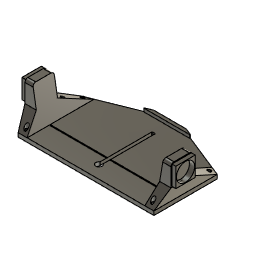
openastrotracker-cameramount (Autodesk Fusion 360 design; units mm, degrees)
Autodesk Fusion 360 part; units mm, degrees
note: some values were not read from the file. Chosen so that the rebuilt part matches the saved one: which bodies a step acts on; which pieces of a blend or face edit are solid.
sketch "Sketch1" plane through (0, 0, 0) normal (0, 1, 0) x (1, 0, 0)
  line L0 (145.5, -42) -> (-145.5, -42)
  line L1 (-145.5, -42) -> (-145.5, 42)
  line L2 (-145.5, 42) -> (145.5, 42)
  line L3 (145.5, 42) -> (145.5, -42)
  line L4 (145.5, -42) -> (-145.5, 42) construction
  line L5 (-145.5, -42) -> (145.5, 42) construction
  dimension "d1" = 291
  dimension "d2" = 84
  constraint perpendicular L0 L1
  constraint parallel L0 L2
  constraint parallel L1 L3
  constraint horizontal L0
  constraint coincident L4 origin
  constraint coincident L5 origin
  measures "d1" distance of L1.end L2.end
  measures "d2" distance of L0.end L1.end
  measures "d167" distance of L0.start
ref_plane "WorkPlane2" through (0, 0, -42) normal (0, 0, 1) x (1, 0, 0)
sketch "Sketch15" plane through (0, 0, -42) normal (0, 0, 1) x (1, 0, 0)
  line L0 (105, 0) -> (105, 95)
  line L1 (105, 95) -> (0, 95)
  line L2 (-105, 0) -> (-105, 95)
  line L3 (-105, 95) -> (0, 95)
  line L4 (105, 0) -> (105, -35)
  line L5 (105, -35) -> (0, -35)
  line L6 (-105, 0) -> (-105, -35)
  line L7 (-105, -35) -> (0, -35)
  line L8 (105, 70) -> (-105, 70)
  line L9 (-105, -20) -> (105, -20)
  line L10 (2.5, 95) -> (-2.5, 95)
  line L11 (-2.5, 95) -> (-2.5, -35)
  line L12 (-2.5, -35) -> (2.5, -35)
  line L13 (2.5, -35) -> (2.5, 95)
  line L14 (2.5, 95) -> (-2.5, -35) construction
  line L15 (-2.5, 95) -> (2.5, -35) construction
  circle A0 centre (0, -15) radius 5
  line L16 (-105, 95) -> (105, 95)
  line L17 (105, 95) -> (105, 90)
  line L18 (105, 90) -> (-105, 90)
  line L19 (-105, 90) -> (-105, 95)
  line L20 (105, 95) -> (-105, 95)
  line L21 (-105, 95) -> (-105, 63)
  line L22 (-105, 63) -> (105, 63)
  line L23 (105, 63) -> (105, 95)
  line L24 (105, 63) -> (25, 95)
  line L25 (-25, 95) -> (-105, 63)
  point P0 (0, 30)
  point P1 (0, 30)
  dimension "d64" = 105
  dimension "d65" = 95
  dimension "d66" = 105
  dimension "d67" = 95
  dimension "d68" = 105
  dimension "d69" = 35
  dimension "d70" = 105
  dimension "d71" = 35
  dimension "d72" = 25
  dimension "d73" = 15
  dimension "d76" = 130
  dimension "d77" = 5
  dimension "d78" = 10
  dimension "d79" = 5
  dimension "d160" = 32
  constraint vertical L0
  constraint horizontal L1
  constraint vertical L2
  constraint horizontal L3
  constraint vertical L4
  constraint horizontal L5
  constraint vertical L6
  constraint horizontal L7
  constraint coincident L0 L8.start
  constraint coincident L2 L8.end
  constraint perpendicular L2 L8
  constraint coincident L6 L9.start
  constraint coincident L4 L9.end
  constraint perpendicular L4 L9
  constraint perpendicular L10 L11
  constraint parallel L10 L12
  constraint parallel L11 L13
  constraint horizontal L10
  constraint coincident L14 P1
  constraint coincident L15 P1
  constraint coincident P1 P0
  constraint horizontal L16
  constraint vertical L17
  constraint horizontal L18
  constraint vertical L19
  constraint horizontal L20
  constraint vertical L21
  constraint horizontal L22
  constraint vertical L23
  constraint coincident L16 L24.end
  constraint coincident L1 L24.end
  constraint coincident L16 L25.start
  measures "d64" distance of origin L0.start
  measures "d65" distance of origin L1.end
  measures "d66" distance of origin L2.start
  measures "d67" distance of origin L1.end
  measures "d68" distance of origin L0.start
  measures "d69" distance of origin L5.end
  measures "d70" distance of origin L2.start
  measures "d71" distance of origin L5.end
  measures "d72" distance of L1 L8
  measures "d73" distance of L7 L9
  measures "d76" distance of L10.end L11.end
  measures "d77" distance of L11.end L12.end
  measures "d78" diameter of A0
  measures "d79" distance of L2.end L18.end
  measures "d160" distance of L0.end L22.end
extrude "Extrude16" add sketch "Sketch15" against normal blind 6 contours L9 L13 A0 | L9 L11 A0 makes body 1 at (2.1131, -19.5315, -46)
extrude "Extrude13" add sketch "Sketch15" against normal blind 6 separate body contours L0 L4 L9 L13 A0 L22 | L0 L8 L23 L24 | L8 L13 L22 L24 | L4 L5 L9 L13 | L0 L8 L18 L23 L24 | L8 L13 L18 L24 | L5 L7 L9 L11 L12 L13 | L0 L1 L16 L17 L18 L20 L23 L24 | L8 L11 L13 L18 | L8 L11 L22 L25 | L2 L6 L9 L11 A0 L22 | L1 L13 L16 L18 L20 L24 | L8 L11 L18 L25 | L1 L3 L10 L11 L13 L16 L18 L20 | L2 L8 L21 L25 | L6 L7 L9 L11 | L2 L8 L18 L21 L25 | L3 L11 L16 L18 L20 L25 | L2 L3 L16 L18 L19 L20 L21 L25 makes body 2
extrude "Extrude14" add sketch "Sketch15" along normal blind 5 contours L0 L1 L16 L17 L18 L20 L23 L24 | L1 L13 L16 L18 L20 L24 | L1 L3 L10 L11 L13 L16 L18 L20 | L3 L11 L16 L18 L20 L25 | L2 L3 L16 L18 L19 L20 L21 L25 bodies 2
sketch "Sketch16" plane through (0, 0, 0) normal (0, 1, 0) x (1, 0, 0)
  line L0 (90, -30) -> (-90, -30)
  line L1 (-90, -30) -> (-90, 30)
  line L2 (-90, 30) -> (90, 30)
  line L3 (90, 30) -> (90, -30)
  line L4 (90, -30) -> (-90, 30) construction
  line L5 (-90, -30) -> (90, 30) construction
  constraint perpendicular L0 L1
  constraint parallel L0 L2
  constraint parallel L1 L3
  constraint horizontal L0
  constraint coincident L4 origin
  constraint coincident L5 origin
extrude "Extrude15" add sketch "Sketch16" along normal blind 10 separate body makes body 3
chamfer "Chamfer6" distance 1 angle 45 2 edges at (2.5, 29.6651, -48) (-2.5, 29.6651, -48) on bodies 2
fillet "Fillet1" radius 1 2 edges at (-2.5, 70, -44.5) (2.5, 70, -44.5) on bodies 2
sketch "Sketch18" plane through (0, 0, -42) normal (0, 0, 1) x (-1, 0, 0)
  line L0 (-105, -90) -> (105, -90)
  line L1 (105, -90) -> (105, 35)
  line L2 (105, 35) -> (-105, 35)
  line L3 (-105, 35) -> (-105, -90)
  arc A0 (-2.5, 19.3301) -> (-2.5, 10.6699) centre (0, 15) ccw
  line L4 (-2.5, 19.3301) -> (-2.5, 20)
  line L5 (-2.5, 20) -> (2.5, 20)
  line L6 (2.5, 20) -> (2.5, 19.3301)
  arc A1 (2.5, 10.6699) -> (2.5, 19.3301) centre (0, 15) ccw
  line L7 (2.5, 10.6699) -> (2.5, -69)
  arc A2 (1.5, -70) -> (2.5, -69) centre (1.5, -69) ccw
  line L8 (1.5, -70) -> (-1.5, -70)
  arc A3 (-2.5, -69) -> (-1.5, -70) centre (-1.5, -69) ccw
  line L9 (-2.5, -69) -> (-2.5, 10.6699)
  line L10 (-105, -90) -> (-92, -90)
  line L11 (-92, -90) -> (-92, 35)
  line L12 (-92, 35) -> (-105, 35)
  line L13 (-105, 35) -> (-105, -90)
  dimension "d93" = 125
  dimension "d94" = 13
  constraint horizontal L10
  constraint vertical L11
  constraint horizontal L12
  constraint vertical L13
  constraint coincident L0.start L3.end
  measures "d93" distance of L0.start L2.end
  measures "d94" distance of L0.start L10.end
extrude "Extrude17" add sketch "Sketch18" along normal blind 5 separate body contours L0 L2 L3 L10 L11 L12 L13 makes body 4
ref_plane "WorkPlane1" through (119, 0, 0) normal (1, 0, 0) x (0, 1, 0)
sketch "Sketch3" plane through (119, 0, 0) normal (1, 0, 0) x (0, 1, 0)
  circle A0 centre (0, 0) radius 14.05
  line L0 (15.01, 15.01) -> (-15.01, 15.01)
  line L1 (-15.01, 15.01) -> (-15.01, -15.01)
  line L2 (-15.01, -15.01) -> (15.01, -15.01)
  line L3 (15.01, -15.01) -> (15.01, 15.01)
  line L4 (15.01, 15.01) -> (-15.01, -15.01) construction
  line L5 (-15.01, 15.01) -> (15.01, -15.01) construction
  dimension "d4" = 28.1
  dimension "d5" = 30.02
  dimension "d6" = 30.02
  constraint coincident A0.centre origin
  constraint perpendicular L0 L1
  constraint parallel L0 L2
  constraint parallel L1 L3
  constraint horizontal L0
  constraint coincident L4 A0.centre
  constraint coincident L5 A0.centre
  measures "d4" diameter of A0
  measures "d5" distance of L0.end L1.end
  measures "d6" distance of L1.end L2.end
extrude "Extrude1" add sketch "Sketch3" against normal blind 20 separate body contours A0 | L0 L1 L2 L3 makes body 5
extrude "Extrude2" cut sketch "Sketch3" against normal blind 8.2 contours A0 bodies 5
extrude "Extrude18" cut 1 faces at (99, -5.0033, 5.0033) along direction (1, 0, 0) blind 5 on bodies 5 bodies 5
extrude "Extrude25" cut 1 faces at (104, -5.0033, 5.0033) along direction (1, 0, 0) blind 1 on bodies 5 bodies 5
sketch "Sketch22" plane through (0, 0, -42) normal (0, 0, 1) x (-1, 0, 0)
  line L0 (-105, -90) -> (105, -90)
  line L1 (105, -90) -> (105, 35)
  line L2 (105, 35) -> (-105, 35)
  line L3 (-105, 35) -> (-105, -90)
  arc A0 (-2.5, 19.3301) -> (-2.5, 10.6699) centre (0, 15) ccw
  line L4 (-2.5, 19.3301) -> (-2.5, 20)
  line L5 (-2.5, 20) -> (2.5, 20)
  line L6 (2.5, 20) -> (2.5, 19.3301)
  arc A1 (2.5, 10.6699) -> (2.5, 19.3301) centre (0, 15) ccw
  line L7 (2.5, 10.6699) -> (2.5, -69)
  arc A2 (1.5, -70) -> (2.5, -69) centre (1.5, -69) ccw
  line L8 (1.5, -70) -> (-1.5, -70)
  arc A3 (-2.5, -69) -> (-1.5, -70) centre (-1.5, -69) ccw
  line L9 (-2.5, -69) -> (-2.5, 10.6699)
  line L10 (-105, -90) -> (-92, -90)
  line L11 (-92, -90) -> (-92, 35)
  line L12 (-92, 35) -> (-105, 35)
  line L13 (-105, 35) -> (-105, -90)
  dimension "d129" = 13
  constraint horizontal L10
  constraint vertical L11
  constraint horizontal L12
  constraint vertical L13
  constraint coincident L0.start L3.end
  measures "d129" distance of L0.start L10.end
extrude "Extrude26" cut 1 faces at (105, -5.0033, 5.0033) along direction (1, 0, 0) blind 8 on bodies 5 bodies 5
sketch "Sketch23" plane through (113, 0, 0) normal (-1, 0, 0) x (0, -1, 0)
  circle A0 centre (0, 0) radius 14.05
  line L0 (-15.01, 15.01) -> (-15.01, -15.01)
  line L1 (-15.01, -15.01) -> (15.01, -15.01)
  line L2 (15.01, -15.01) -> (15.01, 15.01)
  line L3 (15.01, 15.01) -> (-15.01, 15.01)
  line L4 (-16.41, -16.41) -> (16.41, -16.41)
  line L5 (16.41, -16.41) -> (16.41, 16.41)
  line L6 (16.41, 16.41) -> (-16.41, 16.41)
  line L7 (-16.41, 16.41) -> (-16.41, -16.41)
  dimension "d132" = 1.4
extrude "Extrude27" add sketch "Sketch23" along normal blind 22 contours A0 | L0 L1 L2 L3 | L4 L5 L6 L7 bodies 5
extrude "Extrude28" cut 1 faces at (113, -1.8779, -1.8565) along direction (-1, 0, 0) blind 2 on bodies 5 bodies 5
extrude "Extrude35" cut sketch "Sketch15" along normal mid plane 60 contours L0 L8 L23 L24 | L0 L8 L18 L23 L24 | L0 L1 L16 L17 L18 L20 L23 L24 bodies 2
sketch "Sketch29" plane through (0, 0, -42) normal (0, 0, 1) x (-1, 0, 0)
  line L0 (-105, -63) -> (-37.5, -90)
  line L1 (-37.5, -90) -> (105, -90)
  line L2 (105, -90) -> (105, 35)
  line L3 (105, 35) -> (-105, 35)
  line L4 (-105, 35) -> (-105, -63)
  arc A0 (-2.5, 19.3301) -> (-2.5, 10.6699) centre (0, 15) ccw
  line L5 (-2.5, 19.3301) -> (-2.5, 20)
  line L6 (-2.5, 20) -> (2.5, 20)
  line L7 (2.5, 20) -> (2.5, 19.3301)
  arc A1 (2.5, 10.6699) -> (2.5, 19.3301) centre (0, 15) ccw
  line L8 (2.5, 10.6699) -> (2.5, -69)
  arc A2 (1.5, -70) -> (2.5, -69) centre (1.5, -69) ccw
  line L9 (1.5, -70) -> (-1.5, -70)
  arc A3 (-2.5, -69) -> (-1.5, -70) centre (-1.5, -69) ccw
  line L10 (-2.5, -69) -> (-2.5, 10.6699)
  line L11 (-105, 35) -> (-91, 35)
  line L12 (-91, 35) -> (-91, -76.5)
  line L13 (-91, -76.5) -> (-105, -76.5)
  line L14 (-105, -76.5) -> (-105, 35)
  dimension "d163" = 14
  constraint horizontal L11
  constraint vertical L12
  constraint horizontal L13
  constraint vertical L14
  constraint coincident L3.end L4.start
  measures "d163" distance of L3.end L11.end
loft "Loft5" add profiles "Sketch29" section 1 contours L0 L3 L4 L11 L12 L14 section 2 face at (105.6667, 5.47, -16.41) separate body on bodies 5 makes body 6
combine "Combine8" operation add target body 6 tool bodies 5
chamfer "Chamfer11" distance 58.4 distance2 10 1 edges at (91, 0, 16.41) measured on face at (91, 16.67, -33.47) on bodies 6
sketch "Sketch30" plane through (0, 0, -42) normal (0, 0, 1) x (-1, 0, 0)
  line L0 (-105, -63) -> (-37.5, -90)
  line L1 (-37.5, -90) -> (105, -90)
  line L2 (105, -90) -> (105, 35)
  line L3 (105, 35) -> (-105, 35)
  line L4 (-105, 35) -> (-105, -63)
  arc A0 (-2.5, 19.3301) -> (-2.5, 10.6699) centre (0, 15) ccw
  line L5 (-2.5, 19.3301) -> (-2.5, 20)
  line L6 (-2.5, 20) -> (2.5, 20)
  line L7 (2.5, 20) -> (2.5, 19.3301)
  arc A1 (2.5, 10.6699) -> (2.5, 19.3301) centre (0, 15) ccw
  line L8 (2.5, 10.6699) -> (2.5, -69)
  arc A2 (1.5, -70) -> (2.5, -69) centre (1.5, -69) ccw
  line L9 (1.5, -70) -> (-1.5, -70)
  arc A3 (-2.5, -69) -> (-1.5, -70) centre (-1.5, -69) ccw
  line L10 (-2.5, -69) -> (-2.5, 10.6699)
  line L11 (-90, 0.7) -> (90, 0.7)
  line L12 (90, 0.7) -> (90, -0.7)
  line L13 (90, -0.7) -> (-90, -0.7)
  line L14 (-90, -0.7) -> (-90, 0.7)
  line L15 (-90, 0.7) -> (90, -0.7) construction
  line L16 (90, 0.7) -> (-90, -0.7) construction
  dimension "d167" = 180
  dimension "d168" = 1.4
  constraint horizontal L11
  constraint perpendicular L11 L12
  constraint parallel L11 L13
  constraint parallel L12 L14
  constraint coincident L15 origin
  constraint coincident L16 origin
  measures "d167" distance of L12.end L13.end
  measures "d168" distance of L11.end L12.end
extrude "Extrude36" cut sketch "Sketch30" against normal blind 0.6 contours L10 L11 L13 L14 bodies 2
chamfer "Chamfer13" distance 0.4 angle 45 2 edges at (46.25, 0.7, -42.6) (46.25, -0.7, -42.6) on bodies 2
chamfer "Chamfer14" distance 2 angle 45 1 edges at (37.5, 90, -39.5) on bodies 2
sketch "Sketch31" plane through (0, 0, -42) normal (0, 0, -1) x (1, 0, 0)
  line L0 (105, 35) -> (91, 35)
  line L1 (91, 35) -> (91, -68.6)
  line L2 (91, -68.6) -> (105, -63)
  line L3 (105, -63) -> (105, 35)
  circle A0 centre (98, 29) radius 1.7
  circle A1 centre (98, -57.4736) radius 1.7
  circle A2 centre (98, -26.858) radius 1.7
  circle A3 centre (98, 29) radius 2.9
  circle A4 centre (98, -26.858) radius 2.9
  circle A5 centre (98, -57.4736) radius 2.9
  dimension "d173" = 3.4
  dimension "d174" = 6
  dimension "d175" = 3.4
  dimension "d176" = 3.4
  dimension "d177" = 5.8
  dimension "d178" = 5.8
  dimension "d179" = 5.8
  constraint concentric A0 A3
  constraint concentric A2 A4
  constraint concentric A1 A5
  measures "d173" diameter of A0
  measures "d174" distance of L0 A0.centre
  measures "d175" diameter of A1
  measures "d176" diameter of A2
  measures "d177" diameter of A3
  measures "d178" diameter of A4
  measures "d179" diameter of A5
extrude "Extrude37" cut sketch "Sketch31" against normal blind 30 contours A3 | A4 | A5 bodies 6 makes body 7 at (97.5128, 55.8449, -40.216) makes body 8 at (99.6907, 26.6803, -28.4716) makes body 9 at (92.46, 16.6656, -33.4633)
extrude "Extrude38" add sketch "Sketch31" against normal blind 4 contours A3 | A4 | A5 bodies 6 7 8 9
extrude "Extrude39" cut sketch "Sketch31" against normal blind 40 contours A0 | A1 | A2 bodies 6
extrude "Extrude40" cut sketch "Sketch31" along normal blind 9 contours A0 | A1 | A2 bodies 2
fillet "Fillet2" radius 4.5 2 edges at (107, 16.41, 16.41) (107, -16.41, 16.41) on bodies 6
mirror "Mirror8" about plane through (0, 0, 0) normal (1, 0, 0) of bodies 6 makes body 10
delete_face "DeleteFace3" 1 faces at (2.5, -19.7767, -44) on bodies 2
delete_face "DeleteFace4" 1 faces at (-2.5, -19.5534, -44) on bodies 2
split "Split4" by plane through (0, 0, 0) normal (1, 0, 0) bodies 2 makes body 11 at (34.4333, 28.4762, -48)
mirror "Mirror9" about plane through (0, 0, 0) normal (1, 0, 0) of bodies 11 makes body 12
combine "Combine9" operation add target body 12 tool bodies 11
hidden bodies 1 2 4
